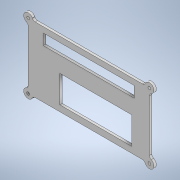
# Autodesk Inventor part: cover_top_v3
Saved by Autodesk Inventor 2022 (Build 260153000, 153)
## iProperties
Created: 2022-08-26
Part Number: cover_top_v3
Material: Generic
Document SubType Name: Modeling
Designer: suerfu
Density: 1 g/cm^3
Appearance: Default
Author: suerfu
Autodesk Inventor part; units mm, degrees
ref_plane "YZ Plane" through (0, 0, 0) normal (1, 0, 0) x (0, 1, 0)
ref_plane "XZ Plane" through (0, 0, 0) normal (0, 1, 0) x (-1, 0, 0)
ref_plane "XY Plane" through (0, 0, 0) normal (0, 0, 1) x (1, 0, 0)
sketch "Sketch1" plane through (0, 0, 0) normal (0, 0, 1) x (1, 0, 0)
  line L0 (-56.2118, 34.29) -> (63.5, 34.29)
  line L1 (63.5, 34.29) -> (63.5, -34.29)
  line L2 (63.5, -34.29) -> (-63.5, -34.29)
  line L3 (-63.5, -34.29) -> (-63.5, 27.0152)
  line L4 (0, 0) -> (-113.7275, 61.4128) construction
  line L5 (-60.325, 31.115) -> (60.325, 31.115)
  line L6 (60.325, 31.115) -> (60.325, -31.115)
  line L7 (60.325, -31.115) -> (-60.325, -31.115)
  line L8 (-60.325, -31.115) -> (-60.325, 31.115)
  circle A0 centre (-63.5, 34.29) radius 4.7625
  line L9 (-59.0352, 35.9473) -> (-59.1884, 36.3601)
  line L10 (-65.4689, 29.9535) -> (-65.5533, 29.9854)
  arc A1 (-63.5, 27.0152) -> (-65.5533, 29.9854) centre (-66.675, 27.0152) ccw
  arc A2 (-59.1884, 36.3601) -> (-56.2118, 34.29) centre (-56.2118, 37.465) ccw
  line L11 (0, 55.5625) -> (0, -55.5625) construction
  line L12 (-104.775, 0) -> (104.775, 0) construction
  circle A3 centre (63.5, 34.29) radius 4.7625
  line L13 (59.0352, 35.9473) -> (59.1884, 36.3601)
  line L14 (65.4689, 29.9535) -> (65.5533, 29.9854)
  arc A4 (65.5533, 29.9854) -> (63.5, 27.0152) centre (66.675, 27.0152) ccw
  arc A5 (56.2118, 34.29) -> (59.1884, 36.3601) centre (56.2118, 37.465) ccw
  line L15 (104.775, 0) -> (-104.775, 0) construction
  circle A6 centre (-63.5, -34.29) radius 4.7625
  line L16 (-59.0352, -35.9473) -> (-59.1884, -36.3601)
  line L17 (-65.4689, -29.9535) -> (-65.5533, -29.9854)
  arc A7 (-65.5533, -29.9854) -> (-63.5, -27.0152) centre (-66.675, -27.0152) ccw
  arc A8 (-56.2118, -34.29) -> (-59.1884, -36.3601) centre (-56.2118, -37.465) ccw
  circle A9 centre (63.5, -34.29) radius 4.7625
  line L18 (65.4689, -29.9535) -> (65.5533, -29.9854)
  arc A10 (63.5, -27.0152) -> (65.5533, -29.9854) centre (66.675, -27.0152) ccw
  line L19 (59.0352, -35.9473) -> (59.1884, -36.3601)
  arc A11 (59.1884, -36.3601) -> (56.2118, -34.29) centre (56.2118, -37.465) ccw
  line L20 (-30.2895, 0.635) -> (45.0215, 0.635)
  line L21 (45.0215, 0.635) -> (45.0215, -27.94)
  line L22 (45.0215, -27.94) -> (-30.2895, -27.94)
  line L23 (-30.2895, -27.94) -> (-30.2895, 0.635)
  line L24 (-47.625, 28.575) -> (47.625, 28.575)
  line L25 (47.625, 28.575) -> (47.625, 17.145)
  line L26 (47.625, 17.145) -> (-47.625, 17.145)
  line L27 (-47.625, 17.145) -> (-47.625, 28.575)
  point P0 (-58.42, 34.29)
  point P1 (-63.5, 29.21)
  point P2 (56.2118, 34.29)
  point P3 (-63.5, -27.0152)
  point P4 (56.2118, -34.29)
  point P5 (63.5, -27.0152)
  point P6 (63.5, 27.0152)
  point P7 (-59.9502, -31.115)
  point P8 (-60.325, -30.7402)
  point P9 (59.9502, -31.115)
  point P10 (60.325, -30.7402)
  point P11 (-60.325, 30.7402)
  point P12 (-59.9502, 31.115)
  point P13 (-66.6527, 30.7204)
  point P14 (-66.6527, -30.7204)
  point P15 (66.6527, -30.7204)
  point P16 (66.6527, 30.7204)
  point P17 (-65.405, 29.9251)
  point P18 (-65.405, -29.9251)
  point P19 (65.405, -29.9251)
  point P20 (65.405, 29.9251)
  dimension "d8" = 63.5
  dimension "d9" = 63.5
  dimension "d10" = 34.29
  dimension "d11" = 34.29
  dimension "d15" = 60.325
  dimension "d16" = 60.325
  dimension "d17" = 62.23
  dimension "d18" = 31.115
  dimension "d19" = 9.525
  dimension "d20" = 5.08
  dimension "d21" = 5.08
  dimension "d22" = 3.175
  dimension "d25" = 48.26
  dimension "d26" = 59.69
  dimension "d27" = 12.7
  dimension "d28" = 107.95
  dimension "d29" = 30.0355
  dimension "d30" = 105.3465
  dimension "d31" = 3.175
  dimension "d32" = 31.75
  constraints: 56 end point, 29 symmetric about line, 24 point on circle, 12 centre point, 8 parallel, 7 point on line, 6 tangent, 5 horizontal, 4 perpendicular, 1 coincident, 1 equal radius, 1 vertical, 9 other
  measures "d8" distance from line of L4.start L3
  measures "d9" distance from line of L1 L4.start
  measures "d10" distance from line of L4.start L2
  measures "d11" distance from line of L0 L4.start
  measures "d15" distance from line of L4.start L8
  measures "d16" distance from line of L4.start L6
  measures "d17" distance between parallel lines of L7 L5
  measures "d18" distance from line of L4.start L5
  measures "d19" diameter of A0
  measures "d20" distance of point (-58.42, 34.29) point (-63.5, 34.29)
  measures "d21" distance of point (-63.5, 34.29) point (-63.5, 29.21)
  measures "d22" radius of A1
  measures "d25" distance between parallel lines of L26 L7
  measures "d26" distance between parallel lines of L24 L7
  measures "d27" distance between parallel lines of L8 L27
  measures "d28" distance between parallel lines of L8 L25
  measures "d29" distance between parallel lines of L8 L23
  measures "d30" distance between parallel lines of L8 L21
  measures "d31" distance between parallel lines of L22 L7
  measures "d32" distance between parallel lines of L20 L7
extrude "Extrusion1" add sketch "Sketch1" along normal blind 2.54
sketch "Sketch2" plane through (0, 0, 2.54) normal (0, 0, 1) x (1, 0, 0)
  circle A0 centre (-63.5, 34.29) radius 2.2451
  circle A1 centre (-63.5, -34.29) radius 1.7045
  circle A2 centre (63.5, 34.29) radius 1.7045
  circle A3 centre (63.5, -34.29) radius 1.5875
  arc A4 (-59.0352, 35.9473) -> (-65.405, 29.9251) centre (-63.5, 34.29) ccw projected
  arc A5 (-65.405, -29.9251) -> (-59.0352, -35.9473) centre (-63.5, -34.29) ccw projected
  arc A6 (65.405, 29.9251) -> (59.0352, 35.9473) centre (63.5, 34.29) ccw projected
  arc A7 (59.0352, -35.9473) -> (65.405, -29.9251) centre (63.5, -34.29) ccw projected
  point P0 (0, 0)
  point P1 (-66.6527, 30.7204)
  point P2 (-66.6527, -30.7204)
  point P3 (66.6527, 30.7204)
  point P4 (66.6527, -30.7204)
  constraints: 4 centre point, 4 coincident, 4 concentric
hole "Hole1" at (-63.5, -34.29, 2.54) at (-63.5, 34.29, 2.54) at (63.5, 34.29, 2.54) at (63.5, -34.29, 2.54) direction (0, 0, -1) diameter 2.9464 end through all clearance for "Socket Head Cap Screw" size "#4" standard "Ansi Unified Screw Threads"
equation "\"d9\" = d8"
equation "\"d11\" = d10"
equation "\"d16\" = d15"
equation "\"d18\" = 0.5 * d17"
equation "\"d20\" = d21"
body "Solid1"
